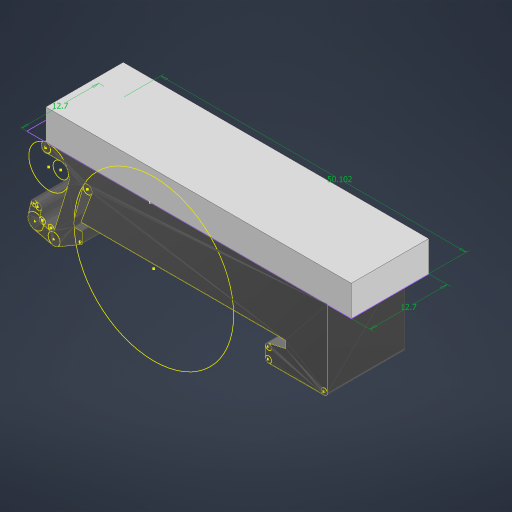
# Autodesk Inventor part: DinRailMount
Saved by Autodesk Inventor 2024 (Build 280153000, 153)
## iProperties
Created: 2025-02-14
Part Number: DinRailMount
Material: Generic
Document SubType Name: Modeling
Designer: Tommy Rohmann
Density: 1 g/cm^3
Appearance: Default
Author: Tommy Rohmann
Autodesk Inventor part; units mm, degrees
ref_plane "YZ Plane" through (0, 0, 0) normal (1, 0, 0) x (0, 1, 0)
ref_plane "XZ Plane" through (0, 0, 0) normal (0, 1, 0) x (-1, 0, 0)
ref_plane "XY Plane" through (0, 0, 0) normal (0, 0, 1) x (1, 0, 0)
sketch "Sketch1" plane through (-17.1345, 0, 0) normal (0, 1, 0) x (-1, 0, 0)
  line L0 (0, 0) -> (-50.1015, 0)
  line L1 (-50.1015, 0) -> (-50.1015, 12.7)
  line L2 (-50.1015, 12.7) -> (0, 12.7)
  line L3 (0, 12.7) -> (0, 0)
  line L4 (0, 0) -> (3.1512, 0)
  line L5 (3.1512, 0) -> (3.1512, 12.7)
  line L6 (3.1512, 12.7) -> (0, 12.7)
  line L7 (0, 12.7) -> (0, 0)
  point P0 (-17.1345, 0)
  dimension "d0" = 12.7
  dimension "d1" = 12.7
  dimension "d2" = 50.1015
  constraints: 16 end point, 4 parallel, 2 horizontal, 2 perpendicular
  measures "d0" distance of L0.end L1.end
  measures "d1" distance of L5.end L4.end
  measures "d2" distance of L0.start L0.end
extrude "Extrusion1" add sketch "Sketch1" along normal blind 5 contours L0 L1 L2 L3
sketch "Sketch2" plane through (-17.1345, 0, 12.7) normal (0, 0, 1) x (1, 0, 0)
  line L0 (-1.1099, -11.3831) -> (-0.7439, -9.8165) projected
  circle A0 centre (-1.2567, -9.7783) radius 0.5081 projected
  line L1 (-1.8863, -9.1095) -> (-1.0637, -9.3017) projected
  circle A1 centre (-1.9245, -9.6223) radius 0.508 projected
  line L2 (-2.4011, -9.4293) -> (-2.9508, -11.7823) projected
  circle A2 centre (-1.7141, -12.0712) radius 1.27 projected
  line L3 (-2.003, -13.3079) -> (1.2722, -14.073) projected
  line L4 (-0.7753, -11.8992) -> (0.8196, -12.2718) projected
  circle A3 centre (-0.5968, -11.4198) radius 0.5079 projected
  circle A4 centre (0.854, -11.7581) radius 0.508 projected
  line L5 (1.3081, -11.9944) -> (3.1279, -5.9557) projected
  circle A5 centre (1.3333, -13.0771) radius 0.9836 projected
  line L6 (1.7634, -13.9605) -> (5.8413, -11.5608) projected
  circle A6 centre (5.6461, -11.4046) radius 0.25 projected
  line L7 (5.8961, -11.4874) -> (5.8961, -9.7282) projected
  line L8 (5.8961, -9.7282) -> (4.6261, -9.7282) projected
  circle A7 centre (17.6977, -9.1402) radius 13.0848 projected
  line L9 (7.558, -3.4083) -> (5.72, -8.4582) projected
  line L10 (4.6261, -8.5522) -> (6.1299, -3.0247) projected
  circle A8 centre (6.8221, -3.2766) radius 0.7366 projected
  line L11 (3.6397, -4.2571) -> (1.3081, -11.9944) projected
  circle A9 centre (0.4781, -3.3043) radius 3.302 projected
  circle A10 centre (2.425, -2.7223) radius 1.27 projected
  line L12 (-0.1284, -1.4523) -> (2.425, -1.4523) projected
  circle A11 centre (0, -0.6903) radius 0.762 projected
  circle A12 centre (0, -0.762) radius 0.762 projected
  line L13 (50.1015, 0) -> (0, 0) projected
  line L14 (46.1627, -12.6573) -> (46.1627, 0) projected
  circle A13 centre (45.6548, -12.5692) radius 0.5079 projected
  line L15 (36.4313, -13.0771) -> (45.7429, -13.0771) projected
  circle A14 centre (36.5107, -12.5691) radius 0.508 projected
  line L16 (36.0027, -10.6927) -> (36.0027, -12.6486) projected
  circle A15 centre (36.5109, -10.7718) radius 0.5082 projected
  line L17 (39.3047, -9.6435) -> (36.3501, -10.2897) projected
  line L18 (39.3047, -8.4582) -> (39.3047, -9.6435) projected
  line L19 (5.72, -8.4582) -> (39.3047, -8.4582) projected
  point P0 (17.1345, 0)
  constraints: 4 other
body "Solid1"
